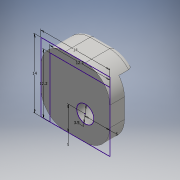
# Autodesk Inventor part: RxBoardMountFoot
Saved by Autodesk Inventor 2016 (Build 200138000, 138)
## iProperties
Created: 2026-04-05
Part Number: RxBoardMountFoot
Material: Generic
Document SubType Name: Modeling
Designer: Steve
Density: 1 g/cm^3
Appearance: Default
Author: Steve
Autodesk Inventor part; units mm, degrees
ref_plane "YZ Plane" through (0, 0, 0) normal (1, 0, 0) x (0, 1, 0)
ref_plane "XZ Plane" through (0, 0, 0) normal (0, 1, 0) x (-1, 0, 0)
ref_plane "XY Plane" through (0, 0, 0) normal (0, 0, 1) x (1, 0, 0)
sketch "Sketch1" plane through (0, 0, 0) normal (0, 1, 0) x (-1, 0, 0)
  line L0 (0, 0) -> (14, 0)
  line L1 (14, 0) -> (14, 14)
  line L2 (14, 14) -> (0, 14)
  line L3 (0, 14) -> (0, 0)
  circle A0 centre (5, 5) radius 1.75
  line L4 (0, 0) -> (12.2, 0)
  line L5 (12.2, 0) -> (12.2, 12.2)
  line L6 (12.2, 12.2) -> (0, 12.2)
  line L7 (0, 12.2) -> (0, 0)
  dimension "d0" = 14
  dimension "d1" = 14
  dimension "d2" = 3.5
  dimension "d3" = 5
  dimension "d4" = 5
  dimension "d5" = 12.2
  dimension "d6" = 12.2
  constraints: 16 end point, 4 parallel, 2 horizontal, 2 perpendicular, 1 centre point
  measures "d0" distance of L2.end L1.end
  measures "d1" distance of L1.end L0.end
  measures "d2" diameter of A0
  measures "d3" distance from line of L0 A0.centre
  measures "d4" distance from line of L3 A0.centre
  measures "d5" distance of L6.end L5.end
  measures "d6" distance of L5.end L4.end
extrude "Extrusion3" add sketch "Sketch1" along normal blind 3 contours L3 L6 L5 L0
extrude "Extrusion4" add sketch "Sketch1" along normal blind 6 contours L5 L6 L3 L2 L1 L0
fillet "Fillet1" radius 5 5 edges at (-14, 3, 0) (-14, 3, 14) (-12.2, 4.5, 12.2) (0, 3, 14) (0, 1.5, 0)
fillet "Fillet2" radius 1 5 edges at (-12.5355, 6, 12.5355) (-7, 6, 14) (-2.8787, 6, 13.5277) (-13.5277, 6, 2.8787) (-14, 6, 7)
body "Solid2"
